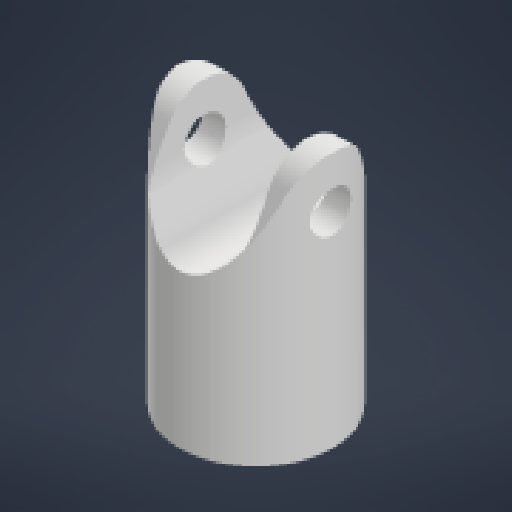
# Autodesk Inventor part: Base_joint
Saved by Autodesk Inventor 2026.2 (Build 302298010, 298A)
## iProperties
Created: 2026-06-25
Part Number: Base_joint
Material: Generic
Document SubType Name: Modeling
Designer: frede
Density: 1 g/cm^3
Appearance: Default
Author: frede
Autodesk Inventor part; units mm, degrees
ref_plane "YZ Plane" through (0, 0, 0) normal (1, 0, 0) x (0, 1, 0)
ref_plane "XZ Plane" through (0, 0, 0) normal (0, 1, 0) x (-1, 0, 0)
ref_plane "XY Plane" through (0, 0, 0) normal (0, 0, 1) x (1, 0, 0)
sketch "Sketch1" plane through (0, 0, 0) normal (0, 1, 0) x (-1, 0, 0)
  circle A0 centre (0, 0) radius 4.925
  arc A1 (3.9454, 1.0194) -> (-3.5041, 2.0801) centre (0, 0) ccw
  line L0 (2.6068, 1.21) -> (3.9454, 1.0194)
  line L1 (2.1655, -1.8895) -> (2.6068, 1.21)
  line L2 (3.5041, -2.0801) -> (2.1655, -1.8895)
  arc A2 (-3.9454, -1.0194) -> (3.5041, -2.0801) centre (0, 0) ccw
  line L3 (-2.6068, -1.21) -> (-3.9454, -1.0194)
  line L4 (-2.1655, 1.8895) -> (-2.6068, -1.21)
  line L5 (-3.5041, 2.0801) -> (-2.1655, 1.8895)
  circle A3 centre (0, 0.038) radius 7.5
  dimension "d4" = 15
  constraints: 12 end point, 4 centre point, 4 point on circle
  measures "d4" diameter of A3
extrude "Extrusion1" add sketch "Sketch1" along normal blind 15 contours A0 | A3
sketch "Sketch2" plane through (0, 15, 0) normal (0, 1, 0) x (1, 0, 0)
  line L0 (-3.9454, -1.0194) -> (-2.6068, -1.21) projected
  line L1 (-2.6068, -1.21) -> (-2.1655, 1.8895) projected
  line L2 (-2.1655, 1.8895) -> (-3.5041, 2.0801) projected
  arc A0 (3.9454, 1.0194) -> (-3.5041, 2.0801) centre (0, 0) ccw projected
  line L3 (3.9454, 1.0194) -> (2.6068, 1.21) projected
  line L4 (2.6068, 1.21) -> (2.1655, -1.8895) projected
  line L5 (2.1655, -1.8895) -> (3.5041, -2.0801) projected
  arc A1 (-3.9454, -1.0194) -> (3.5041, -2.0801) centre (0, 0) ccw projected
  circle A2 centre (0, -0.038) radius 7.5 projected
extrude "Extrusion2" add sketch "Sketch2" along normal blind 10 contours L0 L1 L2 A0 L3 L4 L5 A1 | A2
sketch "Sketch3" plane through (0, 0, 0) normal (1, 0, 0) x (0, 1, 0)
  line L0 (25, -7.462) -> (25, 7.538) projected
  line L1 (0, -7.462) -> (0, 7.538) projected
  line L2 (0, 7.538) -> (25, 7.538) projected
  line L3 (0, -7.462) -> (25, -7.462) projected
  line L4 (25, 0.038) -> (17, 0.038)
  circle A0 centre (21, 0.038) radius 4
  line L5 (25, 7.538) -> (15, 7.538)
  line L6 (15, 7.538) -> (22.7991, 3.6106)
  line L7 (25, -7.462) -> (15, -7.462)
  line L8 (15, -7.462) -> (22.7991, -3.5346)
  point P0 (0, 0)
  dimension "d5" = 8
  dimension "d6" = 10
  dimension "d7" = 10
  constraints: 10 end point, 3 point on circle, 2 midpoint, 2 point on line, 2 tangent, 1 centre point, 1 horizontal
  measures "d5" distance of L4.start L4.end
  measures "d6" distance of L2.end L5.end
  measures "d7" distance of L3.end L7.end
extrude "Extrusion3" cut sketch "Sketch3" along normal mid plane 20 contours L3 L8 A0 L0 | A0 L6 L2 L0
sketch "Sketch4" plane through (0, 0, 0) normal (0, 0, 1) x (1, 0, 0)
  line L0 (6.5944, 22.7991) -> (-6.5944, 22.7991) projected
  line L1 (-6.5944, 22.7991) -> (6.5944, 22.7991) projected
  ellipse E0 centre (0, 29.8935) end of major axis (0, 15) minor radius 7.5 (-6.5944, 22.7991) -> (6.5944, 22.7991) ccw projected
  line L2 (6.5944, 22.7991) -> (-6.5944, 22.7991) projected
  line L3 (7.5, 25) -> (-7.5, 25) projected
  line L4 (-7.5, 0) -> (-7.5, 25) projected
  line L5 (7.5, 0) -> (7.5, 25) projected
  line L6 (0, 25) -> (5, 25)
  line L7 (0, 25) -> (0, 20)
  circle A0 centre (0, 20) radius 5
  line L8 (-5, 25) -> (-5, 20)
  line L9 (5, 20) -> (5, 25)
  point P0 (0, 0)
  point P1 (-4.6939, 18.2775)
  point P2 (4.6939, 18.2775)
  dimension "d10" = 5
  dimension "d11" = 5
  constraints: 8 end point, 3 point on circle, 2 point on line, 2 tangent, 1 centre point, 1 coincident, 1 midpoint, 1 parallel, 1 vertical, 6 other
  measures "d10" distance of L6.start L6.end
  measures "d11" distance of L6.start L7.end
extrude "Extrusion4" cut sketch "Sketch4" along normal mid plane 20 contours L9 A0 L0 | L0 A0 L3 L9 | E0 A0 L0 | L0 L7 A0 | L0 A0 L7 | A0 L0 L8 L3 | A0 L8 L0
sketch "Sketch5" plane through (0, 0, 0) normal (1, 0, 0) x (0, 1, 0)
  line L0 (25, 0.038) -> (20, 0.038)
  line L1 (20, -4.9441) -> (20, 5.0202) projected
  circle A0 centre (20, 0.038) radius 2
  point P0 (0, 0)
  dimension "d16" = 4
  constraints: 2 end point, 1 centre point, 1 midpoint, 2 other
  measures "d16" diameter of A0
extrude "Extrusion5" cut sketch "Sketch5" along normal mid plane 20
body "Solid1"
